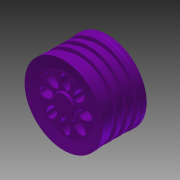
# Autodesk Inventor part: Rueda
Saved by Autodesk Inventor 2014 (Build 180170000, 170)
## iProperties
Created: 2014-01-26
Part Number: Rueda
Material: Plástico ABS
Document SubType Name: Modeling
Designer: Sanjo
Density: 1.06 g/cm^3
Mass: 35.525 g
Surface Area: 80.7006 cm^2
Volume: 33.5141 cm^3
Appearance: Suave - Púrpura
Author: Sanjo
Autodesk Inventor part; units mm, degrees
note: some values were not read from the file. Chosen so that the rebuilt part matches the saved one: direction of "Hole1".
ref_plane "YZ Plane" through (0, 0, 0) normal (1, 0, 0) x (0, 1, 0)
ref_plane "XZ Plane" through (0, 0, 0) normal (0, 1, 0) x (-1, 0, 0)
sketch "Boceto1" plane through (0, 0, 0) normal (1, 0, 0) x (0, 1, 0)
  line L0 (0, 0) -> (-25, 0)
  line L1 (-25, 22.25) -> (-23.898, 16)
  line L2 (-23.898, 16) -> (-23.898, 6)
  line L3 (-25, 22.25) -> (-22.75, 22.25)
  line L4 (-2.25, 22.25) -> (0, 22.25)
  line L5 (-22.75, 22.25) -> (-22.5, 22)
  line L6 (-2.25, 22.25) -> (-2.5, 22)
  line L7 (-25, 0) -> (-25, 5.5)
  line L8 (-24.5, 6) -> (-23.898, 6)
  line L9 (-24.5, 6) -> (-25, 5.5)
  line L10 (0, 22.25) -> (0, 4)
  line L11 (0, 4) -> (5, 4)
  line L12 (5, 4) -> (5, 2)
  line L13 (-4, 2) -> (5, 2)
  line L14 (-4, 2) -> (-4, 0)
  line L15 (-19.375, 22) -> (-19.375, 19.9)
  line L16 (-19.375, 19.9) -> (-16.375, 19.9)
  line L17 (-16.375, 19.9) -> (-16.375, 22)
  line L18 (-13.75, 22) -> (-13.75, 19.9)
  line L19 (-13.75, 19.9) -> (-10.75, 19.9)
  line L20 (-10.75, 19.9) -> (-10.75, 22)
  line L21 (-8.125, 22) -> (-8.125, 19.9)
  line L22 (-8.125, 19.9) -> (-5.125, 19.9)
  line L23 (-5.125, 19.9) -> (-5.125, 22)
  line L24 (-22.5, 22) -> (-19.375, 22)
  line L25 (-16.375, 22) -> (-13.75, 22)
  line L26 (-10.75, 22) -> (-8.125, 22)
  line L27 (-5.125, 22) -> (-2.5, 22)
  point P0 (-25, 2)
  point P1 (-25, 6)
  dimension "d6" = 25
  dimension "d7" = 32
  dimension "d8" = 10
  dimension "d17" = 44.5
  dimension "d18" = 44.5
  dimension "d23" = 0.5
  dimension "d24" = 0.5
  dimension "d31" = 5
  dimension "d32" = 8
  dimension "d41" = 30
  dimension "d42" = 25
  dimension "d45" = 170
  dimension "d56" = 4
  dimension "d60" = 4
  dimension "d61" = 3
  dimension "d62" = 2.625
  dimension "d63" = 2.625
  dimension "d64" = 2.625
  dimension "d66" = 44
  dimension "d67" = 44
  dimension "d68" = 44
  dimension "d69" = 44
  dimension "d70" = 2.1
  constraints: 56 end point, 31 perpendicular, 7 parallel, 5 horizontal, 4 equal length, 4 point on line, 1 vertical, 2 other
  measures "d6" distance of L1.start L4.end
  measures "d7" diameter of L1.end L0
  measures "d8" distance of L1.end L2.end
  measures "d17" diameter of L4 L0
  measures "d18" diameter of L3 L0
  measures "d23" distance of L8.start point (-25, 6)
  measures "d24" distance of L7.end point (-25, 6)
  measures "d31" distance of L10.end L11.end
  measures "d32" diameter of L11 L0
  measures "d41" distance between parallel lines of L7 L12
  measures "d42" distance from line of L7 L0.start
  measures "d45" angle of L2 L1
  measures "d56" diameter of L13 L0
  measures "d60" distance from line of L14 L0.start
  measures "d61" distance of L15.end L16.end
  measures "d62" distance between parallel lines of L17 L18
  measures "d63" distance between parallel lines of L21 L20
  measures "d64" distance from line of L6.end L23
  measures "d66" diameter of L24 L0
  measures "d67" diameter of L25 L0
  measures "d68" diameter of L26 L0
  measures "d69" diameter of L27 L0
  measures "d70" distance between parallel lines of L24 L16
revolve "Revolución1" add sketch "Boceto1" angle 360 about axis through (0, 0, 0) along (0, -1, 0)
sketch "Boceto2" plane through (0, 5, 0) normal (0, 1, 0) x (1, 0, 0)
  circle A0 centre (0, 0) radius 2 projected
  circle A1 centre (0, 0) radius 4 projected
  point P0 (0, -4)
ref_plane "Plano de trabajo1" through (0, 5, 4) normal (0, 0, 1) x (1, 0, 0)
sketch "Boceto3" plane through (0, 5, 4) normal (0, 0, 1) x (1, 0, 0)
  line L0 (22.25, -5) -> (-22.25, -5) projected
  point P0 (0, -5)
  point P1 (0, -2)
  dimension "d33" = 3
  measures "d33" distance from line of L0 point (0, -2)
hole "Hole1" at (0, 3, 4) direction (0, 0, -1) diameter 1.567 end up to surface thread size "M2x0.4" class "6H" standard "ISO Metric profile"
sketch "Boceto4" plane through (0, -23.898, 0) normal (0, -1, 0) x (1, 0, 0)
  ellipse E0 centre (0, 11) end of major axis (1.0353, 7.1363) minor radius 2.5
  dimension "d73" = 4
  dimension "d74" = 2.5
  constraints: 2 other
extrude "Extrusión1" cut sketch "Boceto4" against normal through all
pattern_circular "Patrón circular1" count 8 over 360 about axis through (0, -23.875, 0) along (0, 1, 0) of "Extrusión1"
equation "\"d24\" = d23"
